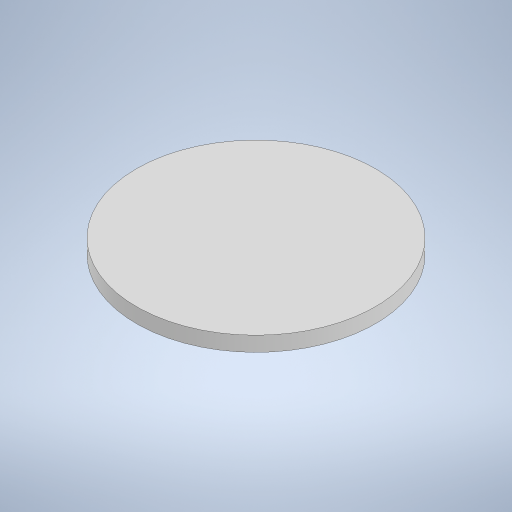
# Autodesk Inventor part: flow director r1
Saved by Autodesk Inventor 2024.1 (Build 281209000, 209)
## iProperties
Created: 2024-08-24
Part Number: flow director r1
Material: Generic
Document SubType Name: Modeling
Designer: pab2
Density: 1 g/cm^3
Appearance: Default
Author: pab2
Autodesk Inventor part; units mm, degrees
ref_plane "YZ Plane" through (0, 0, 0) normal (1, 0, 0) x (0, 1, 0)
ref_plane "XZ Plane" through (0, 0, 0) normal (0, 1, 0) x (-1, 0, 0)
ref_plane "XY Plane" through (0, 0, 0) normal (0, 0, 1) x (1, 0, 0)
sketch "Sketch1" plane through (0, 0, 0) normal (0, 1, 0) x (-1, 0, 0)
  circle A0 centre (0, 0) radius 12.7
  dimension "d0" = 25.4
  constraints: 1 centre point, 1 coincident
  measures "d0" diameter of A0
extrude "Extrusion1" add sketch "Sketch1" along normal blind 1.5748
sketch "Sketch2" plane through (0, 0, 0) normal (0, -1, 0) x (1, 0, 0)
  circle A0 centre (0, 0) radius 9.271
  line L0 (0, -9.271) -> (0, -7.271)
  line L1 (9.271, 0) -> (8.271, 0)
  line L2 (8.271, 0) -> (7.771, 0)
  line L3 (7.771, 0) -> (6.771, 0)
  line L4 (6.771, 0) -> (6.271, 0)
  line L5 (6.271, 0) -> (5.271, 0)
  line L6 (5.271, 0) -> (4.771, 0)
  line L7 (4.771, 0) -> (3.771, 0)
  line L8 (3.771, 0) -> (3.271, 0)
  line L9 (3.271, 0) -> (2.271, 0)
  line L10 (2.271, 0) -> (1.771, 0)
  line L11 (1.771, 0) -> (0.771, 0)
  line L12 (0.771, 0) -> (0.271, 0)
  line L13 (0, 9.271) -> (0, 7.271)
  arc A1 (0, -9.271) -> (0, 9.271) centre (-158.4465, 0) ccw
  arc A2 (0, -9.271) -> (0, 9.271) centre (-55.3547, 0) ccw
  arc A3 (0, -9.271) -> (0, 9.271) centre (-23.3809, 0) ccw
  arc A4 (0, -9.271) -> (0, 9.271) centre (-17.7882, 0) ccw
  arc A5 (0, -9.271) -> (0, 9.271) centre (-11.5029, 0) ccw
  arc A6 (0, -9.271) -> (0, 9.271) centre (-9.5109, 0) ccw
  arc A7 (0, -9.271) -> (0, 9.271) centre (-6.6222, 0) ccw
  arc A8 (0, -9.271) -> (0, 9.271) centre (-5.5177, 0) ccw
  arc A9 (0, -9.271) -> (0, 9.271) centre (-3.7176, 0) ccw
  arc A10 (0, -9.271) -> (0, 9.271) centre (-2.9615, 0) ccw
  arc A11 (0, -9.271) -> (0, 9.271) centre (-1.6448, 0) ccw
  arc A12 (0, -9.271) -> (0, 9.271) centre (-1.0605, 0) ccw
  circle A13 centre (0, 9.271) radius 1
  circle A14 centre (0, -9.271) radius 1
  point P0 (0.974, -9.0443)
  point P1 (0.986, -9.1043)
  point P2 (0.986, 9.1043)
  point P3 (0.974, 9.0443)
  point P4 (0.9357, 8.9182)
  point P5 (0.9084, 8.8528)
  point P6 (0.9084, -8.8528)
  point P7 (0.9357, -8.9182)
  point P8 (0.7874, -8.6546)
  point P9 (0.8347, -8.7203)
  point P10 (0.8347, 8.7203)
  point P11 (0.7874, 8.6546)
  point P12 (0.6008, -8.4716)
  point P13 (0.6706, -8.5292)
  point P14 (0.6706, 8.5292)
  point P15 (0.6008, 8.4716)
  point P16 (0.4399, 8.373)
  point P17 (0.35, 8.3343)
  point P18 (0.35, -8.3343)
  point P19 (0.4399, -8.373)
  point P20 (0.0553, -8.2725)
  point P21 (0.1564, -8.2833)
  point P22 (0.1564, 8.2833)
  point P23 (0.0553, 8.2725)
  dimension "d3" = 18.542
  dimension "d4" = 2
  dimension "d5" = 1
  dimension "d6" = 0.5
  dimension "d7" = 1
  dimension "d8" = 0.5
  dimension "d9" = 1
  dimension "d10" = 0.5
  dimension "d11" = 1
  dimension "d12" = 0.5
  dimension "d13" = 1
  dimension "d14" = 0.5
  dimension "d15" = 1
  dimension "d16" = 0.5
  dimension "d17" = 2
  dimension "d18" = 2
  dimension "d19" = 2
  constraints: 39 point on circle, 28 end point, 15 centre point, 11 point on line, 3 coincident, 2 vertical, 1 horizontal
  measures "d3" diameter of A0
  measures "d4" distance of L0.start L0.end
  measures "d5" distance of L1.start L1.end
  measures "d6" distance of L1.end L2.end
  measures "d7" distance of L2.end L3.end
  measures "d8" distance of L3.end L4.end
  measures "d9" distance of L4.end L5.end
  measures "d10" distance of L5.end L6.end
  measures "d11" distance of L6.end L7.end
  measures "d12" distance of L7.end L8.end
  measures "d13" distance of L8.end L9.end
  measures "d14" distance of L9.end L10.end
  measures "d15" distance of L10.end L11.end
  measures "d16" distance of L11.end L12.end
  measures "d17" distance of L13.start L13.end
  measures "d18" diameter of A13
  measures "d19" diameter of A14
extrude "Extrusion2" add sketch "Sketch2" along normal blind 1.8 contours A12 A14 A11 L2 | L2 A11 A13 A12 | A13 A2 L12 A1 | A13 A4 L10 A3 | A13 A6 L8 A5 | A13 A8 L6 A7 | A13 A10 L4 A9 | A1 L12 A2 A14 | A3 L10 A4 A14 | A5 L8 A6 A14 | A7 L6 A8 A14 | A9 L4 A10 A14
mirror "Mirror1" about plane through (0, 0, 0) normal (1, 0, 0) of "Extrusion2"
body "Solid1"
